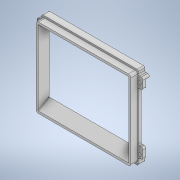
# Autodesk Inventor part: DisplayBezel
Saved by Autodesk Inventor 2020 (Build 240168000, 168)
## iProperties
Created: 2021-07-04
Part Number: DisplayBezel
Material: Generic
Document SubType Name: Modeling
Designer: 10300812
Density: 1 g/cm^3
Appearance: Default
Author: 10300812
Autodesk Inventor part; units mm, degrees
ref_plane "YZ Plane" through (0, 0, 0) normal (1, 0, 0) x (0, 1, 0)
ref_plane "XZ Plane" through (0, 0, 0) normal (0, 1, 0) x (-1, 0, 0)
ref_plane "XY Plane" through (0, 0, 0) normal (0, 0, 1) x (1, 0, 0)
sketch "Sketch1" plane through (0, 0, 0) normal (0, 0, 1) x (1, 0, 0)
  line L0 (-81.5, 70) -> (81.5, 70)
  line L1 (81.5, 70) -> (81.5, -70)
  line L2 (81.5, -70) -> (-81.5, -70)
  line L3 (-81.5, -70) -> (-81.5, 70)
  line L4 (-81.5, 70) -> (81.5, -70) construction
  line L5 (81.5, 70) -> (-81.5, -70) construction
  line L6 (81.5, 62) -> (89.5, 62)
  line L7 (89.5, 62) -> (89.5, 44)
  line L8 (89.5, 44) -> (81.5, 44)
  line L9 (81.5, 44) -> (81.5, 62)
  line L10 (81.5, -58) -> (89.5, -58)
  line L11 (89.5, -58) -> (89.5, -40)
  line L12 (89.5, -40) -> (81.5, -40)
  line L13 (81.5, -40) -> (81.5, -58)
  line L14 (-81.5, 62) -> (-89.5, 62)
  line L15 (-89.5, 62) -> (-89.5, 44)
  line L16 (-89.5, 44) -> (-81.5, 44)
  line L17 (-81.5, 44) -> (-81.5, 62)
  line L18 (-81.5, -58) -> (-89.5, -58)
  line L19 (-89.5, -58) -> (-89.5, -40)
  line L20 (-89.5, -40) -> (-81.5, -40)
  line L21 (-81.5, -40) -> (-81.5, -58)
  point P0 (0, 0)
  dimension "d0" = 163
  dimension "d1" = 140
  dimension "d2" = 8
  dimension "d3" = 18
  dimension "d4" = 8
  dimension "d5" = 12
  constraints: 44 end point, 10 parallel, 10 point on line, 5 horizontal, 5 perpendicular, 2 collinear, 2 midpoint
  measures "d0" distance of L0.start L0.end
  measures "d1" distance of L0.end L1.end
  measures "d2" distance of L6.start L6.end
  measures "d3" distance of L6.end L7.end
  measures "d4" distance from line of L14.end L0
  measures "d5" distance between parallel lines of L2 L10
extrude "Extrusion1" add sketch "Sketch1" along normal blind 5
sketch "Sketch2" plane through (0, 0, 5) normal (0, 0, 1) x (1, 0, 0)
  line L0 (-80, -67) -> (80, -67)
  line L1 (80, -67) -> (80, 67)
  line L2 (80, 67) -> (-80, 67)
  line L3 (-80, 67) -> (-80, -67)
  line L4 (-80, -67) -> (80, 67) construction
  line L5 (80, -67) -> (-80, 67) construction
  line L6 (81.5, 70) -> (-81.5, 70) projected
  line L7 (81.5, -40) -> (81.5, 44) projected
  point P0 (0, 0)
  dimension "d48" = 160
  dimension "d49" = 134
  constraints: 12 end point, 2 midpoint, 2 parallel, 1 horizontal, 1 perpendicular
  measures "d48" distance of L1.end L2.end
  measures "d49" distance of L2.end L0.start
extrude "Extrusion2" add sketch "Sketch2" along normal blind 11
sketch "Sketch3" plane through (0, 0, 0) normal (1, 0, 0) x (0, 1, 0)
  line L0 (49.75, 0) -> (-49.75, 0)
  line L1 (49.75, 0) -> (66.532, 20)
  line L2 (66.532, 20) -> (-66.532, 20)
  line L3 (-66.532, 20) -> (-49.75, 0)
  point P0 (0, 0)
  point P1 (0, 0)
  dimension "d12" = 99.5
  dimension "d13" = 20
  dimension "d14" = 130
  dimension "d15" = 130
  constraints: 8 end point, 2 horizontal, 1 coincident, 1 midpoint
  measures "d12" distance of L0.start L0.end
  measures "d13" distance between parallel lines of L0 L2
  measures "d14" angle of L1 L0
  measures "d15" angle of L3 L0
extrude "Extrusion3" cut sketch "Sketch3" against normal mid plane 148
chamfer "Chamfer1" distance 2.82 angle 80 1 edges at (74, 0, 16) measured on face at (74.5, 0, 16)
chamfer "Chamfer2" distance 2.82 angle 80 1 edges at (-74, 0, 16) measured on face at (-74.5, 0, 16)
fillet "Fillet1" radius 4 4 edges at (-80, 67, 10.5) (-80, -67, 10.5) (80, 67, 10.5) (80, -67, 10.5)
fillet "Fillet3" radius 1 4 edges at (-75.41, -56.4657, 8.0035) (75.41, -56.4657, 8.0035) (75.41, 56.4657, 8.0035) (-75.41, 56.4657, 8.0035)
fillet "Fillet4" radius 3 8 edges at (89.5, 62, 2.5) (89.5, -40, 2.5) (89.5, -58, 2.5) (89.5, 44, 2.5) (-89.5, 62, 2.5) (-89.5, 44, 2.5) (-89.5, -40, 2.5) (-89.5, -58, 2.5)
fillet "Fillet5" radius 2 12 edges at (-81.5, 70, 2.5) (81.5, 70, 2.5) (-81.5, -70, 2.5) (81.5, -70, 2.5) (-81.5, -58, 2.5) (-81.5, 44, 2.5) (81.5, -40, 2.5) (81.5, -58, 2.5) (81.5, 62, 2.5) (-81.5, 62, 2.5) (-81.5, -40, 2.5) (81.5, 44, 2.5)
sketch "Sketch4" plane through (0, 0, 5) normal (0, 0, 1) x (1, 0, 0)
  line L0 (-84, -50.9) -> (84, -50.9)
  line L1 (84, -50.9) -> (84, 50.9)
  line L2 (84, 50.9) -> (-84, 50.9)
  line L3 (-84, 50.9) -> (-84, -50.9)
  line L4 (-84, -50.9) -> (84, 50.9) construction
  line L5 (84, -50.9) -> (-84, 50.9) construction
  line L6 (-89.5, 59) -> (-89.5, 47) projected
  line L7 (89.5, 47) -> (89.5, 59) projected
  line L8 (89.5, -55) -> (89.5, -43) projected
  line L9 (-89.5, -43) -> (-89.5, -55) projected
  line L10 (76, 67) -> (-76, 67) projected
  point P0 (0, 0)
  point P1 (-84, 52.5)
  point P2 (84, 53)
  point P3 (84, -52)
  point P4 (-84, -49.5)
  point P5 (89.5, 53)
  dimension "d30" = 168
  dimension "d38" = 102
  dimension "d39" = 101.8
  dimension "d50" = 14.5
  constraints: 12 end point, 4 vertical alignment, 3 midpoint, 2 parallel, 1 horizontal, 1 horizontal alignment, 1 perpendicular
  measures "d30" distance of L0.start L0.end
  measures "d38" distance of point (-84, -49.5) point (-84, 52.5)
  measures "d39" distance of L0.end L1.end
  measures "d50" distance from line of point (-84, 52.5) L10
hole "Hole1" at (-84, 52.5, 5) at (84, 53, 5) at (84, -52, 5) at (-84, -49.5, 5) direction (0, 0, -1) diameter 5.2 end through all
sketch "Sketch5" plane through (0, 0, 0) normal (0, 0, -1) x (-1, 0, 0)
  line L0 (-96.4, 58.75) -> (96.4, 58.75)
  line L1 (96.4, 58.75) -> (96.4, -58.75)
  line L2 (96.4, -58.75) -> (-96.4, -58.75)
  line L3 (-96.4, -58.75) -> (-96.4, 58.75)
  line L4 (-96.4, 58.75) -> (96.4, -58.75) construction
  line L5 (96.4, 58.75) -> (-96.4, -58.75) construction
  circle A0 centre (-84, -52) radius 2.6 projected
  circle A1 centre (84, 52.5) radius 2.6 projected
  circle A2 centre (-84, 53) radius 2.6 projected
  circle A3 centre (84, -49.5) radius 2.6 projected
  line L6 (-74, -49.75) -> (-74, 49.75) projected
  line L7 (-74, 49.75) -> (74, 49.75) projected
  line L8 (74, 49.75) -> (74, -49.75) projected
  line L9 (74, -49.75) -> (-74, -49.75) projected
  arc A4 (-81.5, -68) -> (-79.5, -70) centre (-79.5, -68) ccw projected
  line L10 (79.5, -70) -> (-79.5, -70) projected
  arc A5 (79.5, -70) -> (81.5, -68) centre (79.5, -68) ccw projected
  line L11 (81.5, -60) -> (81.5, -68) projected
  arc A6 (83.5, -58) -> (81.5, -60) centre (83.5, -60) ccw projected
  line L12 (86.5, -58) -> (83.5, -58) projected
  arc A7 (86.5, -58) -> (89.5, -55) centre (86.5, -55) ccw projected
  line L13 (89.5, -43) -> (89.5, -55) projected
  arc A8 (89.5, -43) -> (86.5, -40) centre (86.5, -43) ccw projected
  line L14 (83.5, -40) -> (86.5, -40) projected
  arc A9 (81.5, -38) -> (83.5, -40) centre (83.5, -38) ccw projected
  line L15 (81.5, 42) -> (81.5, -38) projected
  arc A10 (83.5, 44) -> (81.5, 42) centre (83.5, 42) ccw projected
  line L16 (86.5, 44) -> (83.5, 44) projected
  arc A11 (86.5, 44) -> (89.5, 47) centre (86.5, 47) ccw projected
  line L17 (89.5, 59) -> (89.5, 47) projected
  arc A12 (89.5, 59) -> (86.5, 62) centre (86.5, 59) ccw projected
  line L18 (83.5, 62) -> (86.5, 62) projected
  arc A13 (81.5, 64) -> (83.5, 62) centre (83.5, 64) ccw projected
  line L19 (81.5, 68) -> (81.5, 64) projected
  arc A14 (81.5, 68) -> (79.5, 70) centre (79.5, 68) ccw projected
  line L20 (-79.5, 70) -> (79.5, 70) projected
  arc A15 (-79.5, 70) -> (-81.5, 68) centre (-79.5, 68) ccw projected
  line L21 (-81.5, 64) -> (-81.5, 68) projected
  arc A16 (-83.5, 62) -> (-81.5, 64) centre (-83.5, 64) ccw projected
  line L22 (-86.5, 62) -> (-83.5, 62) projected
  arc A17 (-86.5, 62) -> (-89.5, 59) centre (-86.5, 59) ccw projected
  line L23 (-89.5, 47) -> (-89.5, 59) projected
  arc A18 (-89.5, 47) -> (-86.5, 44) centre (-86.5, 47) ccw projected
  line L24 (-83.5, 44) -> (-86.5, 44) projected
  arc A19 (-81.5, 42) -> (-83.5, 44) centre (-83.5, 42) ccw projected
  line L25 (-81.5, -38) -> (-81.5, 42) projected
  arc A20 (-83.5, -40) -> (-81.5, -38) centre (-83.5, -38) ccw projected
  line L26 (-86.5, -40) -> (-83.5, -40) projected
  arc A21 (-86.5, -40) -> (-89.5, -43) centre (-86.5, -43) ccw projected
  line L27 (-89.5, -55) -> (-89.5, -43) projected
  arc A22 (-89.5, -55) -> (-86.5, -58) centre (-86.5, -55) ccw projected
  line L28 (-83.5, -58) -> (-86.5, -58) projected
  arc A23 (-81.5, -60) -> (-83.5, -58) centre (-83.5, -60) ccw projected
  line L29 (-81.5, -68) -> (-81.5, -60) projected
  point P0 (0, 0)
  point P1 (89.458, -58.5)
  point P2 (-89.458, -58.5)
  point P3 (-89.5, 58.75)
  point P4 (89.5, 58.75)
  point P5 (81.9388, -58.75)
  point P6 (-81.9388, -58.75)
  dimension "d40" = 192.8
  dimension "d41" = 117.5
  constraints: 12 end point, 2 midpoint, 2 parallel, 1 horizontal, 1 perpendicular
  measures "d40" distance of L1.end L2.end
  measures "d41" distance of L0.end L1.end
extrude "Extrusion4" add sketch "Sketch5" along normal blind 6 contours L23 A17 L22 A16 L21 A15 L20 A14 L19 A13 L18 A12 L17 L0 | L2 A6 L11 A5 L10 A4 L29 A23
sketch "Sketch6" plane through (0, 0, -6) normal (0, 0, -1) x (-1, 0, 0)
  line L0 (81.9388, -58.75) -> (-81.9388, -58.75) projected
  line L1 (-35, -58.75) -> (35, -58.75)
  line L2 (35, -58.75) -> (35, -61.75)
  line L3 (35, -61.75) -> (-35, -61.75)
  line L4 (-35, -61.75) -> (-35, -58.75)
  point P0 (0, 0)
  point P1 (89.458, -58.5)
  point P2 (-89.458, -58.5)
  point P3 (0, -58.75)
  point P4 (35, -58.5)
  dimension "d44" = 3
  dimension "d45" = 70
  constraints: 8 end point, 2 parallel, 1 horizontal, 1 midpoint, 1 perpendicular, 3 other
  measures "d44" distance of L3.end L1.start
  measures "d45" distance of L2.end L3.end
extrude "Extrusion5" cut sketch "Sketch6" against normal up to surface (6 mm away)
body "Solid1"
